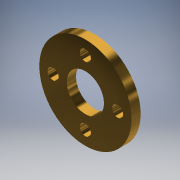
# Autodesk Inventor part: JTW20
Saved by Autodesk Inventor 2019.4 (Build 234330000, 330)
## iProperties
Created: 2019-12-31
Part Number: JTW20
Material: Brass, Soft Yellow
Document SubType Name: Modeling
Designer: Mark
Mass: 64.7923 g
Surface Area: 45.3954 cm^2
Volume: 7.64962 cm^3
Density: 8.47 g/cm^3
Appearance: Brass - Satin
Author: Mark
Autodesk Inventor part; units mm, degrees
ref_plane "YZ Plane" through (0, 0, 0) normal (1, 0, 0) x (0, 1, 0)
ref_plane "XZ Plane" through (0, 0, 0) normal (0, 1, 0) x (-1, 0, 0)
ref_plane "XY Plane" through (0, 0, 0) normal (0, 0, 1) x (1, 0, 0)
sketch "Sketch1" plane through (0, 0, 0) normal (0, 0, 1) x (1, 0, 0)
  circle A0 centre (0, 0) radius 10.1
  circle A1 centre (0, 0) radius 25
  circle A2 centre (0, 0) radius 17.5 construction
  circle A3 centre (0, 17.5) radius 3
  circle A4 centre (-17.5, 0) radius 3
  circle A5 centre (0, -17.5) radius 3
  circle A6 centre (17.5, 0) radius 3
  line L0 (0, 0) -> (0, 17.5)
  line L1 (0, 0) -> (17.5, 0) construction
  dimension "d0" = 20.2
  dimension "d1" = 50
  dimension "d2" = 35
  dimension "d3" = 6
  dimension "d6" = 360
  dimension "d8" = 90
  constraints: 7 centre point, 4 coincident, 4 end point, 2 point on circle, 1 horizontal, 1 perpendicular, 9 other
  measures "d0" diameter of A0
  measures "d1" diameter of A1
  measures "d2" diameter of A2
  measures "d3" diameter of A3
  measures "d8" angle of L1 L0
extrude "Extrusion1" add sketch "Sketch1" along normal blind 5
body "Solid1"
